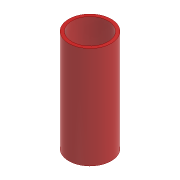
# Autodesk Inventor part: servo shaft spacer short
Saved by Autodesk Inventor 2020 (Build 240168000, 168)
## iProperties
Created: 2020-01-05
Part Number: servo shaft spacer short
Material: Generic
Document SubType Name: Modeling
Designer: ball
Density: 1 g/cm^3
Appearance: Default
Author: ball
Autodesk Inventor part; units mm, degrees
ref_plane "YZ Plane" through (0, 0, 0) normal (1, 0, 0) x (0, 1, 0)
ref_plane "XZ Plane" through (0, 0, 0) normal (0, 1, 0) x (-1, 0, 0)
ref_plane "XY Plane" through (0, 0, 0) normal (0, 0, 1) x (1, 0, 0)
sketch "Sketch1" plane through (0, 0, 0) normal (0, 1, 0) x (-1, 0, 0)
  circle A0 centre (0, 0) radius 3.3655
  circle A1 centre (0, 0) radius 3.937
  dimension "d0" = 6.731
  dimension "d1" = 7.874
  constraints: 2 centre point, 2 coincident
  measures "d0" diameter of A0
  measures "d1" diameter of A1
extrude "Extrusion1" add sketch "Sketch1" along normal blind 18.923
body "Solid1"
